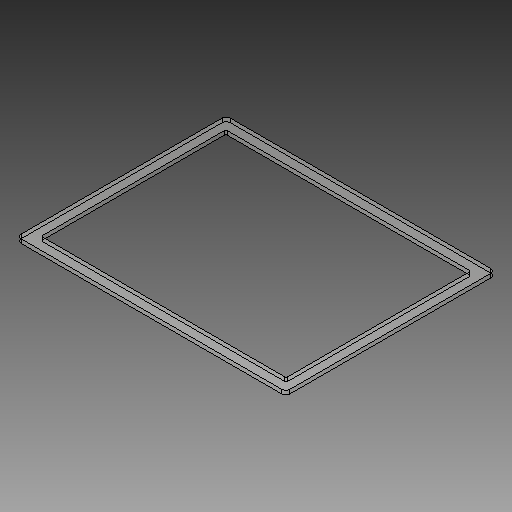
# Autodesk Inventor part: frame_upper
Saved by Autodesk Inventor 2017 (Build 210142000, 142)
## iProperties
Created: 2017-04-26
Part Number: frame_upper
Material: Tworzywo sztuczne PMMA
Document SubType Name: Modeling
Designer: Speed King
Density: 1.188 g/cm^3
Appearance: Poliwęglan — przezroczysty
Mass: 103.475 g
Surface Area: 461.899 cm^2
Volume: 87.0999 cm^3
Author: Speed King
Autodesk Inventor part; units mm, degrees
ref_plane "YZ Plane" through (0, 0, 0) normal (1, 0, 0) x (0, 1, 0)
ref_plane "XZ Plane" through (0, 0, 0) normal (0, 1, 0) x (-1, 0, 0)
ref_plane "XY Plane" through (0, 0, 0) normal (0, 0, 1) x (1, 0, 0)
sketch "Szkic1" plane through (0, 0, 0) normal (0, 1, 0) x (-1, 0, 0)
  line L0 (-169, -131.5) -> (169, -131.5)
  line L1 (169, -131.5) -> (169, 131.5)
  line L2 (169, 131.5) -> (-169, 131.5)
  line L3 (-169, 131.5) -> (-169, -131.5)
  line L4 (-169, -131.5) -> (169, 131.5) construction
  line L5 (169, -131.5) -> (-169, 131.5) construction
  point P0 (0, 0)
  dimension "d0" = 338
  dimension "d1" = 263
  constraints: 12 end point, 2 midpoint, 2 parallel, 1 horizontal, 1 perpendicular
  measures "d0" distance of L2.end L1.end
  measures "d1" distance of L1.end L0.end
extrude "Wyciągnięcie proste1" add sketch "Szkic1" along normal blind 5
sketch "Szkic2" plane through (0, 0, 0) normal (0, -1, 0) x (1, 0, 0)
  line L0 (154, -116) -> (-154, -116)
  line L1 (-154, -116) -> (-154, 116)
  line L2 (-154, 116) -> (154, 116)
  line L3 (154, 116) -> (154, -116)
  line L4 (154, -116) -> (-154, 116) construction
  line L5 (-154, -116) -> (154, 116) construction
  point P0 (0, 0)
  dimension "d4" = 308
  dimension "d5" = 232
  constraints: 12 end point, 2 midpoint, 2 parallel, 1 horizontal, 1 perpendicular
  measures "d4" distance of L1.end L2.end
  measures "d5" distance of L0.end L1.end
extrude "Wyciągnięcie proste2" cut sketch "Szkic2" against normal blind 10
fillet "Zaokrąglenie1" radius 2 4 edges at (-154, 2.5, 116) (-154, 2.5, -116) (154, 2.5, 116) (154, 2.5, -116)
fillet "Zaokrąglenie2" radius 5 4 edges at (169, 2.5, -131.5) (-169, 2.5, -131.5) (169, 2.5, 131.5) (-169, 2.5, 131.5)
